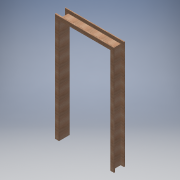
# Autodesk Inventor part: Rahmen
Saved by Autodesk Inventor 2017 (Build 210142000, 142)
## iProperties
Created: 2017-06-02
Part Number: Rahmen
Material: Holz (Birke)
Document SubType Name: Modeling
Designer: Fake
Density: 0.55 g/cm^3
Appearance: Birke - natur - poliert
Author: Fake
Autodesk Inventor part; units mm, degrees
ref_plane "YZ Plane" through (0, 0, 0) normal (1, 0, 0) x (0, 1, 0)
ref_plane "XZ Plane" through (0, 0, 0) normal (0, 1, 0) x (-1, 0, 0)
ref_plane "XY Plane" through (0, 0, 0) normal (0, 0, 1) x (1, 0, 0)
sketch "Skizze1" plane through (0, 0, 0) normal (0, 1, 0) x (-1, 0, 0)
  line L0 (475, 920) -> (-475, 920) construction
  line L1 (-475, 920) -> (-475, -980) construction
  line L2 (475, -980) -> (475, 920) construction
  line L3 (749, 0) -> (-749, 0) projected
  line L4 (0, -1372) -> (0, 1372) projected
  line L5 (535, 980) -> (-535, 980)
  line L6 (-535, 980) -> (-535, -980)
  line L7 (535, -980) -> (535, 980)
  line L8 (-535, -980) -> (-475, -980)
  line L9 (475, -980) -> (535, -980)
  line L10 (460, 905) -> (-460, 905)
  line L11 (-460, 905) -> (-460, -980)
  line L12 (460, -980) -> (460, 905)
  line L13 (-475, -980) -> (-460, -980)
  line L14 (460, -980) -> (475, -980)
  dimension "d0" = 1900
  dimension "d1" = 950
  dimension "d2" = 60
  dimension "d3" = 60
  dimension "d4" = 60
  dimension "d7" = 15
  dimension "d8" = 15
  dimension "d9" = 15
  constraints: 28 end point, 7 parallel, 4 collinear, 3 horizontal, 3 perpendicular, 2 other
  measures "d0" distance of L2.start L0.start
  measures "d1" distance between parallel lines of L1 L2
  measures "d2" distance between parallel lines of L2 L7
  measures "d3" distance between parallel lines of L1 L6
  measures "d4" distance between parallel lines of L0 L5
  measures "d7" distance between parallel lines of L2 L12
  measures "d8" distance between parallel lines of L11 L1
  measures "d9" distance between parallel lines of L0 L10
extrude "Extrusion1" add sketch "Skizze1" along normal blind 20 contours L7 L9 L14 L12 L3 | L3 L12 L10 L4 L5 L7 | L4 L10 L11 L3 L6 L5 | L11 L13 L8 L6 L3
sketch "Skizze2" plane through (0, 20, 0) normal (0, 1, 0) x (1, 0, 0)
  line L0 (-535, -980) -> (535, -980) projected
  line L1 (535, -980) -> (535, 980) projected
  line L2 (535, 980) -> (460, 980) projected
  line L3 (460, 980) -> (460, -905) projected
  line L4 (460, -905) -> (-460, -905) projected
  line L5 (-460, -905) -> (-460, 980) projected
  line L6 (-460, 980) -> (-535, 980) projected
  line L7 (-535, 980) -> (-535, -980) projected
  line L8 (535, 980) -> (460, 980) projected
  line L9 (475, 980) -> (475, -920)
  line L10 (475, -920) -> (-475, -920)
  line L11 (-475, -920) -> (-475, 980)
  line L12 (0, 1372) -> (0, -1372) projected
  line L13 (-749, 0) -> (749, 0) projected
  line L14 (460, 980) -> (460, -905) projected
  line L15 (475, 980) -> (460, 980)
  line L16 (460, -905) -> (-460, -905) projected
  line L17 (460, 980) -> (460, -905)
  line L18 (460, -905) -> (-460, -905)
  line L19 (-460, -905) -> (-460, 980)
  line L20 (-460, 980) -> (-535, 980) projected
  line L21 (-475, 980) -> (-460, 980)
  dimension "d10" = 950
  dimension "d11" = 1900
  constraints: 16 end point, 4 perpendicular, 2 horizontal, 2 point on line, 1 collinear, 1 vertical, 1 other
  measures "d10" distance of L9.end L10.end
  measures "d11" distance between parallel lines of L2 L10
extrude "Extrusion2" add sketch "Skizze2" along normal blind 100 contours L12 L4 L3 L13 L9 L10 | L10 L11 L13 L5 L4 L12 | L11 L6 L5 L13 | L13 L3 L2 L9
chamfer "Fase1" distance 5 angle 45 6 edges at (-460, 0, -37.5) (0, 0, 905) (460, 0, -37.5) (0, 0, 980) (535, 0, 0) (-535, 0, 0)
mirror "Spiegeln1" about plane through (0, 120, 150.1399) normal (0, 1, 0) of "Extrusion1", "Extrusion2", "Fase1"
equation "\"d3\" = d2"
equation "\"d4\" = d2"
